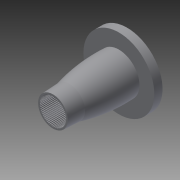
# Autodesk Inventor part: Cable end at actuator
Saved by Autodesk Inventor 2014 SP2 (Build 180246200, 246)
## iProperties
Created: 2015-10-09
Part Number: Cable end at actuator
Material: Generic
Document SubType Name: Modeling
Designer: Lukasz Szmit
Density: 1 g/cm^3
Appearance: Default
Author: Lukasz Szmit
Autodesk Inventor part; units mm, degrees
sketch "Sketch1" plane through (0, 0, 0) normal (0, 1, 0) x (-1, 0, 0)
  circle A0 centre (0, 0) radius 10.75
  dimension "d0" = 21.5
  constraints: 1 centre point, 1 coincident
  measures "d0" diameter of A0
extrude "Extrusion1" add sketch "Sketch1" against normal blind 2.5
ref_plane "Work Plane1" through (0, -22.5, 0) normal (0, -1, 0) x (1, 0, 0)
sketch "Sketch9" plane through (0, -22.5, 0) normal (0, -1, 0) x (1, 0, 0)
  circle A0 centre (0, 0) radius 4.5
  dimension "d9" = 9
  constraints: 1 centre point, 1 coincident
  measures "d9" diameter of A0
ref_plane "Work Plane3" through (0, -2.5, 0) normal (0, -1, 0) x (1, 0, 0)
sketch "Sketch10" plane through (0, -2.5, 0) normal (0, -1, 0) x (1, 0, 0)
  circle A0 centre (0, 0) radius 10.75 construction
  circle A1 centre (0, 0) radius 6.25
  dimension "d12" = 12.5
  constraints: 1 centre point, 1 coincident
  measures "d12" diameter of A1
ref_plane "Work Plane4" through (0, -12.5, 0) normal (0, -1, 0) x (1, 0, 0)
sketch "Sketch11" plane through (0, -12.5, 0) normal (0, -1, 0) x (1, 0, 0)
  circle A0 centre (0, 0) radius 5.75
  dimension "d14" = 11.5
  constraints: 1 centre point, 1 coincident
  measures "d14" diameter of A0
ref_plane "Work Plane5" through (0, -17.5, 0) normal (0, -1, 0) x (1, 0, 0)
sketch "Sketch12" plane through (0, -17.5, 0) normal (0, -1, 0) x (1, 0, 0)
  circle A0 centre (0, 0) radius 4.75
  dimension "d16" = 9.5
  constraints: 1 centre point, 1 coincident
  measures "d16" diameter of A0
loft "Loft1" add profiles "Sketch10", "Sketch11", "Sketch12"
loft "Loft2" add profiles "Sketch9" section 1 edges at (-4.75, -17.5, 0)
sketch "Sketch14" plane through (0, -22.5, 0) normal (0, -1, 0) x (1, 0, 0)
  point P0 (0, 0)
  point P1 (0, 0)
  constraints: 1 coincident
hole "Hole1" at (0, -22.5, 0) direction (0, 1, 0) diameter 3 end through all counterbore diameter 8 counterbore depth 20
ref_plane "Work Plane6" through (0, -11.25, 0) normal (0, -1, 0) x (1, 0, 0)
sketch "Sketch17" plane through (0, -22.5, 0) normal (0, -1, 0) x (1, 0, 0)
  circle A0 centre (0, 0) radius 4 construction
  spline S0 degree 3 poles (5.5421, 2.0819) (5.8131, 1.3603) (5.9407, 0.5926) (5.8943, -0.9485) (5.7209, -1.7072) (5.0929, -3.1153) (4.6444, -3.7513) (3.5289, -4.8156) (2.8725, -5.2337) (1.4364, -5.7948) (0.6705, -5.9324) (-0.8711, -5.9063) (-1.632, -5.7428) (-3.0482, -5.1334) (-3.69, -4.6933) (-4.7689, -3.5918) (-5.1956, -2.9409) (-5.7754, -1.5124) (-5.9231, -0.7483) (-5.9172, 0.7935) (-5.7637, 1.5565) (-5.1729, 2.9806) (-4.7413, 3.6281) (-3.654, 4.7213) (-3.0089, 5.1565) (-1.588, 5.7551) (-0.8259, 5.9128) (0.7158, 5.9271) (1.4807, 5.7836) (2.9124, 5.2116) (3.5656, 4.7885) (4.4328, 3.9484) (4.7117, 3.6109) (5.1903, 2.8809) (5.3886, 2.4905) (5.5421, 2.0819) knots 0 0 0 0 0.231269 0.231269 0.462539 0.462539 0.693808 0.693808 0.925077 0.925077 1.156346 1.156346 1.387616 1.387616 1.618885 1.618885 1.850154 1.850154 2.081423 2.081423 2.312693 2.312693 2.543962 2.543962 2.775231 2.775231 3.0065 3.0065 3.23777 3.23777 3.469039 3.469039 3.599981 3.599981 3.730924 3.730924 3.730924 3.730924 construction
  line L0 (-0.1023, 3.9987) -> (-0.026, 3.8487)
  line L1 (0.0223, 3.8488) -> (0.0977, 3.9988)
  arc A1 (-0.026, 3.8487) -> (0.0223, 3.8488) centre (-0.0019, 3.861) ccw
  arc A2 (0.0977, 3.9988) -> (-0.1023, 3.9987) centre (0, 0) ccw
  dimension "d59" = 0.15
  dimension "d60" = 0.15
  dimension "d61" = 0.2
  dimension "d62" = 4
  constraints: 6 point on circle, 4 end point, 3 centre point, 2 tangent, 1 coincident, 1 other
  measures "d59" vertical distance of L1.start L1.end
  measures "d60" vertical distance of L0.start L0.end
  measures "d61" distance of L1.end L0.start
  measures "d62" radius of A2
extrude "Extrusion2" add sketch "Sketch17" against normal blind 20
pattern_circular "Circular Pattern2" count 60 over 360 about axis through (0, -10, 0) along (0, 1, 0) of "Extrusion2"
equation "\"d60\" = d59"
body "Solid1"
